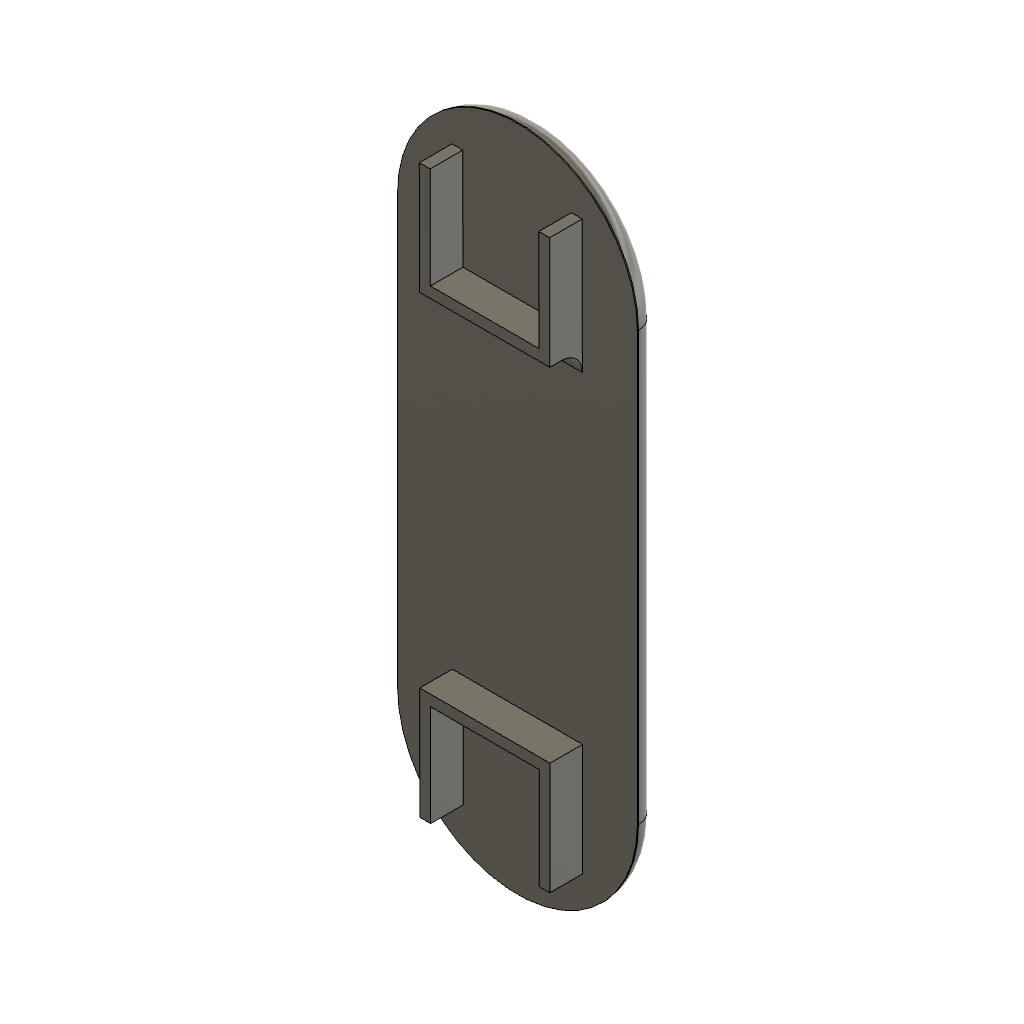
top plate (couvercle) (Autodesk Fusion 360 design; units mm, degrees)
part number: 2026-09-30-11-21-08-868
Autodesk Fusion 360 part; units mm, degrees
sketch "Boceto1" plane through (0, 0, 0) normal (0, 0, 1) x (1, 0, 0)
  line L0 (37.3693, 70) -> (37.3693, 30.5735)
  line L1 (15.2693, 30.5734) -> (15.2693, 69.9734)
  arc A0 (15.2693, 30.5734) -> (37.3693, 30.5735) centre (26.3193, 30.5735) ccw
  arc A1 (37.3693, 70) -> (15.2693, 69.9734) centre (26.3193, 70) ccw
  line L2 (20.3193, 24.17) -> (20.3193, 34.5)
  line L3 (20.3193, 34.5) -> (32.3193, 34.5)
  line L4 (32.3193, 34.5) -> (32.3193, 24.17)
  line L5 (32.3193, 24.17) -> (31.3193, 24.17)
  line L6 (31.3193, 24.17) -> (31.3193, 33.5)
  line L7 (31.3193, 33.5) -> (21.3193, 33.5)
  line L8 (21.3193, 33.5) -> (21.3193, 24.17)
  line L9 (21.3193, 24.17) -> (20.3193, 24.17)
  line L10 (15.2693, 30.5734) -> (15.2693, 50.2734)
  line L11 (20.2878, 76.3829) -> (20.3003, 66.0529)
  line L12 (20.3003, 66.0529) -> (32.3002, 66.0673)
  line L13 (32.3002, 66.0673) -> (32.2878, 76.3973)
  line L14 (32.2878, 76.3973) -> (31.2878, 76.3961)
  line L15 (31.2878, 76.3961) -> (31.299, 67.0661)
  line L16 (31.299, 67.0661) -> (21.2991, 67.0541)
  line L17 (21.2991, 67.0541) -> (21.2878, 76.3841)
  line L18 (21.2878, 76.3841) -> (20.2878, 76.3829)
  dimension "d1" = 39.4
  dimension "d2" = 22.1
  dimension "d11" = 1
  dimension "d12" = 1
  dimension "d13" = 10
  dimension "d14" = 12
  dimension "d15" = 10.33
  dimension "d16" = 1
  dimension "d25" = 10.33
  constraint vertical L0
  constraint vertical L1
  constraint tangent L0 A1
  constraint tangent L0 A0
  constraint vertical L2
  constraint perpendicular L2 L3
  constraint perpendicular L3 L4
  constraint perpendicular L4 L5
  constraint perpendicular L5 L6
  constraint perpendicular L6 L7
  constraint perpendicular L7 L8
  constraint perpendicular L2 L9
  constraint midpoint L1 L10.end
  measures "d1" distance of L1.end L1.start
  measures "d2" distance of L0.end L1.start
  measures "d11" distance of L2.start L8.end
  measures "d12" distance of L4.end L5.end
  measures "d13" distance of L6.end L7.end
  measures "d14" distance of L2.end L3.end
  measures "d15" distance of L3.end L4.end
  measures "d16" distance of L3 L7.end
  measures "d25" distance of L2.start L2.end
extrude "Extruir2" add sketch "Boceto1" along normal blind 5 contours L11 L12 L13 L14 L15 L16 L17 L18 makes body 1
extrude "Extruir3" add sketch "Boceto1" along normal blind 5 separate body contours L2 L3 L4 L5 L6 L7 L8 L9 makes body 2
extrude "Extruir4" add sketch "Boceto1" along normal blind 2 bodies 1 2
fillet "Empalme2" radius 1.9 5 edges at (26.3003, 66.0601, 2) (15.2693, 50.2734, 0) (26.3193, 19.5235, 0) (37.3693, 50.2867, 0) (26.306, 81.05, 0) on bodies 1
named bodies: "top plate with support for springs"
